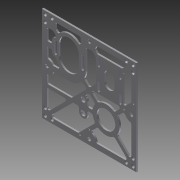
# Autodesk Inventor part: upper gearbox top plate
Saved by Autodesk Inventor 2012 (Build 160160000, 160)
## iProperties
Created: 2012-07-07
Part Number: upper gearbox top plate
Material: Default
Document SubType Name: Modeling
Designer: Bryce
Density: 1 g/cm^3
Author: Bryce
Autodesk Inventor part; units mm, degrees
ref_plane "YZ Plane" through (0, 0, 0) normal (1, 0, 0) x (0, 1, 0)
ref_plane "XZ Plane" through (0, 0, 0) normal (0, 1, 0) x (-1, 0, 0)
ref_plane "XY Plane" through (0, 0, 0) normal (0, 0, 1) x (1, 0, 0)
sketch "Sketch1" plane through (0, 0, 0) normal (0, 0, 1) x (1, 0, 0)
  line L0 (-114.3, 114.3) -> (63.5, 114.3)
  line L1 (63.5, 114.3) -> (63.5, -28.575)
  line L2 (63.5, -63.5) -> (28.575, -63.5)
  line L3 (-114.3, -63.5) -> (-114.3, 114.3)
  circle A0 centre (6.35, -6.35) radius 17.4625
  circle A1 centre (44.45, 107.95) radius 1.5875
  circle A2 centre (-95.25, -57.15) radius 1.5875
  circle A3 centre (-107.95, 95.25) radius 1.5875
  circle A4 centre (-107.95, 107.95) radius 1.5875
  circle A5 centre (-95.25, 107.95) radius 1.5875
  circle A6 centre (57.15, 95.25) radius 1.5875
  circle A7 centre (-107.95, -57.15) radius 1.5875
  circle A8 centre (-107.95, -44.45) radius 1.5875
  circle A9 centre (57.15, 107.95) radius 1.5875
  circle A10 centre (-63.5, 73.025) radius 19.05
  circle A11 centre (-63.5, 53.975) radius 19.05
  line L4 (-82.55, 73.025) -> (-44.45, 73.025)
  line L5 (-44.45, 73.025) -> (-44.45, 53.975)
  line L6 (-44.45, 53.975) -> (-82.55, 53.975)
  line L7 (-82.55, 53.975) -> (-82.55, 73.025)
  arc A12 (-13.7147, 9.2246) -> (-18.8508, -3.175) centre (6.35, -6.35) ccw
  arc A13 (26.4147, -21.9246) -> (26.4147, 9.2246) centre (6.35, -6.35) ccw
  arc A14 (-9.2246, -26.4147) -> (21.9246, -26.4147) centre (6.35, -6.35) ccw
  arc A15 (21.9246, 13.7147) -> (-9.2246, 13.7147) centre (6.35, -6.35) ccw
  arc A16 (-63.3483, 22.2254) -> (-38.6735, 34.1834) centre (-63.5, 53.975) ccw
  line L8 (53.975, 104.775) -> (53.975, 45.7651)
  line L9 (53.975, -53.975) -> (49.4849, -53.975) construction
  line L10 (-104.775, -53.975) -> (-104.775, -49.4849) construction
  line L11 (-63.3483, 22.2254) -> (-92.4782, 22.2254)
  line L12 (21.9246, -26.4147) -> (36.7849, -41.275)
  line L13 (26.4147, -21.9246) -> (41.275, -36.7849)
  line L14 (-13.7147, -21.9246) -> (-45.7651, -53.975)
  line L15 (-9.2246, -26.4147) -> (-24.1468, -41.337)
  line L16 (-13.7147, 9.2246) -> (-25.4, 20.9099)
  line L17 (-9.2246, 13.7147) -> (-20.9099, 25.4)
  line L18 (26.4147, 9.2246) -> (41.337, 24.1468)
  line L19 (21.9246, 13.7147) -> (36.7849, 28.575)
  arc A17 (-35.1635, 39.6536) -> (-31.75, 53.975) centre (-63.5, 53.975) ccw
  line L20 (53.975, -49.4849) -> (53.975, -53.975) construction
  line L21 (49.4849, -53.975) -> (36.7849, -53.975)
  line L22 (-45.7651, -53.975) -> (-100.2849, -53.975)
  line L23 (-104.775, -53.975) -> (-60.325, -9.525) construction
  line L24 (-104.775, -49.4849) -> (-64.8151, -9.525)
  line L25 (53.975, 104.775) -> (38.1, 88.9) construction
  line L26 (53.975, 100.2849) -> (38.1, 84.4099)
  line L27 (49.4849, 104.775) -> (36.7849, 92.075)
  line L28 (-58.4651, -3.175) -> (-29.8901, 25.4)
  line L29 (-29.8901, 25.4) -> (-38.6735, 34.1834)
  line L30 (-25.4, 29.8901) -> (-35.1635, 39.6536)
  line L31 (-18.8508, -3.175) -> (-28.751, -3.175)
  line L32 (-104.775, -9.525) -> (-64.8151, -9.525)
  line L33 (-58.4651, -3.175) -> (-104.775, -3.175)
  arc A18 (-18.8508, -9.525) -> (-13.7147, -21.9246) centre (6.35, -6.35) ccw
  line L34 (-55.8349, -9.525) -> (-100.2849, -53.975)
  line L35 (-49.4849, -3.175) -> (-34.0583, 12.2516) construction
  line L36 (36.7849, -53.975) -> (-12.7, -53.975)
  line L37 (53.975, -36.7849) -> (53.975, -49.4849)
  line L38 (41.275, -36.7849) -> (53.975, -49.4849)
  line L39 (36.7849, -41.275) -> (49.4849, -53.975)
  line L40 (28.575, -63.5) -> (-114.3, -63.5)
  line L41 (63.5, -28.575) -> (63.5, -63.5)
  line L42 (-25.4, -53.975) -> (-25.4, -63.5) construction
  circle A19 centre (44.45, -57.15) radius 1.5875
  circle A20 centre (57.15, -57.15) radius 1.5875
  circle A21 centre (57.15, -44.45) radius 1.5875
  line L43 (6.35, -6.35) -> (-25.0809, -37.7809) construction
  line L44 (-43.0414, -55.7414) -> (-50.8, -63.5) construction
  line L45 (-25.0809, -37.7809) -> (-43.0414, -55.7414) construction
  line L46 (6.35, -6.35) -> (40.026, 27.326) construction
  line L47 (40.026, 27.326) -> (57.9865, 45.2865) construction
  line L48 (57.9865, 45.2865) -> (63.5, 50.8) construction
  arc A22 (-12.7, -53.975) -> (-24.1468, -41.337) centre (-25.4, -53.975) ccw
  arc A23 (41.337, 24.1468) -> (53.975, 12.7) centre (53.975, 25.4) ccw
  line L49 (53.975, 12.7) -> (53.975, -36.7849)
  arc A24 (-31.75, 93.7765) -> (-19.808, 93.3724) centre (-25.4, 104.775) ccw
  line L50 (-31.75, 93.7765) -> (-31.75, 53.975)
  line L51 (-12.7, 104.775) -> (53.975, 104.775)
  arc A25 (-104.775, 12.7) -> (-92.4782, 22.2254) centre (-104.775, 25.4) ccw
  line L52 (-91.44, 53.975) -> (-86.36, 53.975)
  line L53 (-86.36, 53.975) -> (-86.36, 73.025)
  line L54 (-86.36, 73.025) -> (-91.44, 73.025)
  line L55 (-91.44, 73.025) -> (-91.44, 53.975)
  arc A26 (-86.36, 73.025) -> (-91.44, 73.025) centre (-88.9, 73.025) ccw
  arc A27 (-91.44, 53.975) -> (-86.36, 53.975) centre (-88.9, 53.975) ccw
  line L56 (-40.64, 53.975) -> (-35.56, 53.975)
  line L57 (-35.56, 53.975) -> (-35.56, 73.025)
  line L58 (-35.56, 73.025) -> (-40.64, 73.025)
  line L59 (-40.64, 73.025) -> (-40.64, 53.975)
  arc A28 (-35.56, 73.025) -> (-40.64, 73.025) centre (-38.1, 73.025) ccw
  arc A29 (-40.64, 53.975) -> (-35.56, 53.975) centre (-38.1, 53.975) ccw
  line L60 (-36.6885, -17.4625) -> (6.35, -6.35) construction
  line L61 (-36.6885, 4.7625) -> (6.35, -6.35) construction
  line L62 (6.35, -6.35) -> (-104.775, -6.35) construction
  arc A30 (-28.751, 4.7625) -> (-34.0583, 12.2516) centre (-36.6885, 4.7625) ccw
  line L63 (-28.751, 4.7625) -> (-28.751, -3.175)
  arc A31 (-44.626, -17.4625) -> (-28.751, -17.4625) centre (-36.6885, -17.4625) ccw
  line L64 (-44.626, -9.525) -> (-44.626, -17.4625)
  line L65 (-28.751, -17.4625) -> (-28.751, -9.525)
  line L66 (-55.8349, -9.525) -> (-44.626, -9.525)
  line L67 (-28.751, -9.525) -> (-18.8508, -9.525)
  line L68 (-28.751, -3.175) -> (-49.4849, -3.175) construction
  line L69 (-34.0583, 12.2516) -> (-25.4, 20.9099)
  arc A32 (-9.7028, 74.295) -> (-5.5372, 74.295) centre (-7.62, 74.295) ccw
  line L70 (-5.5372, 74.295) -> (-9.7028, 74.295)
  line L71 (-9.7028, 74.295) -> (-9.7028, 86.995)
  arc A33 (-5.5372, 86.995) -> (-9.7028, 86.995) centre (-7.62, 86.995) ccw
  circle A34 centre (12.7, 66.675) radius 9.525
  line L72 (3.175, 66.675) -> (22.225, 66.675)
  line L73 (22.225, 66.675) -> (22.225, 53.975)
  circle A35 centre (12.7, 53.975) radius 9.525
  line L74 (3.175, 53.975) -> (3.175, 66.675)
  line L75 (22.225, 53.975) -> (3.175, 53.975)
  line L76 (-9.7028, 86.995) -> (-5.5372, 86.995)
  line L77 (-5.5372, 86.995) -> (-5.5372, 74.295)
  line L78 (30.9372, 74.295) -> (30.9372, 86.995)
  arc A36 (35.1028, 86.995) -> (30.9372, 86.995) centre (33.02, 86.995) ccw
  line L79 (35.1028, 86.995) -> (35.1028, 74.295)
  line L80 (35.1028, 74.295) -> (30.9372, 74.295)
  arc A37 (30.9372, 74.295) -> (35.1028, 74.295) centre (33.02, 74.295) ccw
  line L81 (-9.7028, 33.655) -> (-9.7028, 46.355)
  arc A38 (-5.5372, 46.355) -> (-9.7028, 46.355) centre (-7.62, 46.355) ccw
  line L82 (-5.5372, 46.355) -> (-5.5372, 33.655)
  line L83 (-5.5372, 33.655) -> (-9.7028, 33.655)
  arc A39 (-9.7028, 33.655) -> (-5.5372, 33.655) centre (-7.62, 33.655) ccw
  line L84 (30.9372, 33.655) -> (30.9372, 46.355)
  arc A40 (35.1028, 46.355) -> (30.9372, 46.355) centre (33.02, 46.355) ccw
  line L85 (35.1028, 46.355) -> (35.1028, 33.655)
  line L86 (35.1028, 33.655) -> (30.9372, 33.655)
  arc A41 (30.9372, 33.655) -> (35.1028, 33.655) centre (33.02, 33.655) ccw
  line L87 (-12.7, 92.075) -> (-10.3326, 92.075) construction
  line L88 (38.1, 92.075) -> (38.1, 84.4099) construction
  line L89 (36.7849, 28.575) -> (-17.7349, 28.575)
  line L90 (-12.7, 92.075) -> (-12.7, 85.0797) construction
  line L91 (-25.4, 104.775) -> (12.7, 60.325) construction
  line L92 (38.1, 84.4099) -> (38.1, 29.8901)
  line L93 (36.7849, 92.075) -> (38.1, 92.075) construction
  line L94 (-19.808, 93.3724) -> (-12.7, 85.0797)
  line L95 (-14.9868, 97.5049) -> (-10.3326, 92.075)
  line L96 (-10.3326, 92.075) -> (36.7849, 92.075)
  line L97 (-12.7, 85.0797) -> (-12.7, 42.5901)
  arc A42 (-19.808, 93.3724) -> (-14.9868, 97.5049) centre (-25.4, 104.775) ccw construction
  arc A43 (-14.9868, 97.5049) -> (-12.7, 104.775) centre (-25.4, 104.775) ccw
  line L98 (-25.4, 29.8901) -> (-12.7, 42.5901)
  line L99 (-20.9099, 25.4) -> (-17.7349, 28.575)
  line L100 (36.7849, 28.575) -> (38.1, 29.8901) construction
  line L101 (38.1, 29.8901) -> (53.975, 45.7651)
  arc A44 (-88.1063, 47.6748) -> (-75.7974, 31.7504) centre (-63.5, 53.975) ccw
  line L102 (-75.7974, 31.7504) -> (-93.7767, 31.7504)
  arc A45 (-93.7767, 31.7504) -> (-104.775, 38.1) centre (-104.775, 25.4) ccw
  line L103 (-104.775, 38.1) -> (-104.775, 57.15)
  line L104 (-104.775, 57.15) -> (-95.25, 57.15)
  line L105 (-95.25, 57.15) -> (-95.25, 53.975)
  arc A46 (-95.25, 53.975) -> (-88.1063, 47.6748) centre (-88.9, 53.975) ccw
  line L106 (-104.775, 88.9) -> (-93.3901, 88.9)
  line L107 (-104.775, 88.9) -> (-104.775, 66.675)
  line L108 (-104.775, 66.675) -> (-95.25, 66.675)
  line L109 (-95.25, 66.675) -> (-95.25, 73.025)
  line L110 (-114.3, 114.3) -> (63.5, -63.5) construction
  arc A47 (-87.0446, 82.5545) -> (-88.1063, 79.3252) centre (-63.5, 73.025) ccw
  arc A48 (-88.1063, 79.3252) -> (-95.25, 73.025) centre (-88.9, 73.025) ccw
  line L111 (-93.3901, 88.9) -> (-87.0446, 82.5545)
  line L112 (-88.9, 104.775) -> (-88.9, 93.3901)
  line L113 (-88.9, 93.3901) -> (-83.8006, 88.2908)
  arc A49 (-41.275, 85.3217) -> (-83.8006, 88.2908) centre (-63.5, 73.025) ccw
  line L114 (-41.275, 85.3217) -> (-41.275, 104.775)
  line L115 (-88.9, 104.775) -> (-41.275, 104.775)
  line L116 (-104.775, -49.4849) -> (-104.775, 12.7)
  line L117 (-100.2849, -53.975) -> (-104.775, -53.975) construction
  point P0 (0, 0)
  point P1 (-88.9, 63.5)
  point P2 (-38.1, 63.5)
  point P3 (3.175, 60.325)
  point P4 (12.7, 66.675)
  dimension "d87" = 38.1
  dimension "d89" = 38.1
  dimension "d309" = 19.05
  dimension "d310" = 19.05
  dimension "d0" = 114.3
  dimension "d1" = 177.8
  dimension "d2" = 177.8
  dimension "d3" = 114.3
  dimension "d4" = 34.925
  dimension "d5" = 57.15
  dimension "d6" = 57.15
  dimension "d10" = 3.175
  dimension "d12" = 3.175
  dimension "d15" = 6.35
  dimension "d16" = 19.05
  dimension "d19" = 6.35
  dimension "d20" = 19.05
  dimension "d23" = 3.175
  dimension "d24" = 6.35
  dimension "d25" = 19.05
  dimension "d26" = 3.175
  dimension "d27" = 6.35
  dimension "d28" = 6.35
  dimension "d29" = 6.35
  dimension "d30" = 19.05
  dimension "d34" = 3.175
  dimension "d35" = 6.35
  dimension "d36" = 6.35
  dimension "d37" = 6.35
  dimension "d38" = 19.05
  dimension "d39" = 3.175
  dimension "d40" = 3.175
  dimension "d47" = 3.175
  dimension "d48" = 6.35
  dimension "d49" = 6.35
  dimension "d50" = 3.175
  dimension "d51" = 19.05
  dimension "d52" = 6.35
  dimension "d88" = 41.275
  dimension "d91" = 50.8
  dimension "d95" = 19.05
  dimension "d98" = 25.4
  dimension "d99" = 25.4
  dimension "d140" = 25.4
  dimension "d141" = 25.4
  dimension "d142" = 25.4
  dimension "d143" = 25.4
  dimension "d167" = 9.525
  dimension "d168" = 9.525
  dimension "d169" = 31.75
  dimension "d171" = 158.75
  dimension "d172" = 158.75
  dimension "d173" = 9.525
  dimension "d174" = 9.525
  dimension "d177" = 92.0746
  dimension "d180" = 45
  dimension "d182" = 6.35
  dimension "d183" = 6.35
  dimension "d186" = 6.35
  dimension "d188" = 6.35
  dimension "d190" = 3.175
  dimension "d195" = 3.175
  dimension "d197" = 3.175
  dimension "d198" = 6.35
  dimension "d204" = 3.175
  dimension "d205" = 3.175
  dimension "d206" = 6.35
  dimension "d207" = 3.175
  constraints: 238 end point, 71 point on circle, 70 parallel, 46 centre point, 42 perpendicular, 25 point on line, 21 coincident, 15 collinear, 13 tangent, 10 horizontal, 6 horizontal alignment, 4 midpoint, 4 vertical alignment, 3 symmetric about line, 3 vertical, 56 other
  measures "d0" distance from line of L0 point (0, 0)
  measures "d1" distance of L0.end L2.start
  measures "d2" distance of L0.start L0.end
  measures "d3" distance from line of L3 point (0, 0)
  measures "d4" diameter of A0
  measures "d5" distance from line of L1 A0.centre
  measures "d6" distance from line of L2 A0.centre
  measures "d10" diameter of A1
  measures "d12" diameter of A2
  measures "d15" distance from line of L0 A1.centre
  measures "d16" distance from line of L1 A1.centre
  measures "d19" distance from line of L2 A2.centre
  measures "d20" distance from line of L3 A2.centre
  measures "d23" diameter of A3
  measures "d24" distance from line of L3 A3.centre
  measures "d25" distance from line of L0 A3.centre
  measures "d26" diameter of A4
  measures "d27" distance from line of L0 A4.centre
  measures "d28" distance from line of L3 A4.centre
  measures "d29" distance from line of L0 A5.centre
  measures "d30" distance from line of L3 A5.centre
  measures "d34" diameter of A9
  measures "d35" distance from line of L0 A9.centre
  measures "d36" distance from line of L1 A9.centre
  measures "d37" distance from line of L1 A6.centre
  measures "d38" distance from line of L0 A6.centre
  measures "d39" diameter of A6
  measures "d40" diameter of A5
  measures "d47" diameter of A7
  measures "d48" distance from line of L2 A7.centre
  measures "d49" distance from line of L3 A7.centre
  measures "d50" diameter of A8
  measures "d51" distance from line of L2 A8.centre
  measures "d52" distance from line of L3 A8.centre
  measures "d88" distance from line of L0 point (-63.5, 73.025)
  measures "d91" distance from line of point (-63.5, 53.975) L3
  measures "d95" distance of L6.end L4.start
  measures "d98" horizontal distance of point (-63.5, 53.975) point (-88.9, 63.5)
  measures "d99" horizontal distance of point (-38.1, 63.5) point (-63.5, 73.025)
  measures "d140" radius of A13
  measures "d141" radius of A14
  measures "d142" radius of A12
  measures "d143" radius of A15
  measures "d167" distance from line of L4 point (-88.9, 63.5)
  measures "d168" distance from line of L4 point (-38.1, 63.5)
  measures "d169" radius of A16
  measures "d171" distance of L9.start L23.start
  measures "d172" distance of L8.start L9.start
  measures "d173" distance between parallel lines of L2 L9
  measures "d174" distance between parallel lines of L1 L8
  measures "d177" distance between parallel lines of L0 L11
  measures "d180" angle of L9 L12
  measures "d182" distance between parallel lines of L13 L12
  measures "d183" distance between parallel lines of L14 L15
  measures "d186" distance between parallel lines of L17 L16
  measures "d188" distance between parallel lines of L19 L18
  measures "d190" distance from line of L14 A0.centre
  measures "d195" distance between parallel lines of L24 L23
  measures "d197" distance between parallel lines of L27 L25
  measures "d198" distance between parallel lines of L26 L27
  measures "d204" distance from line of A0.centre L31
  measures "d205" distance from line of A0.centre L32
  measures "d206" distance between parallel lines of L32 L33
  measures "d207" distance between parallel lines of L34 L23
extrude "Extrusion8" add sketch "Sketch1" along normal blind 3.175 contours L0 L1 L41 L2 L40 L3 | L55 L54 L53 L52 | L52 A27 | A26 L54 | L59 L58 L57 L56 | L56 A29 | A28 L58 | L70 A32 | L71 L76 L77 L70 | A33 L76 | L72 A34 | L73 A35 A34 | A34 A35 L72 | A34 A35 L74 | A35 L75 A34 | A34 A35 | A35 L75 | L78 A36 L79 L80 | L80 A37 | L81 A38 L82 L83 | L83 A39 | L84 A40 L85 L86 | L86 A41 | A44 L102 A45 L103 L104 L105 A46 | L106 L111 A47 A48 L109 L108 L107 | L115 L114 A49 L113 L112
fillet "Fillet3" radius 3.175 31 edges at (21.9246, -26.4147, 1.5875) (49.4849, -53.975, 1.5875) (53.975, -49.4849, 1.5875) (-9.2246, -26.4147, 1.5875) (26.4147, 9.2246, 1.5875) (26.4147, -21.9246, 1.5875) (-18.8508, -9.525, 1.5875) (-9.2246, 13.7147, 1.5875) (21.9246, 13.7147, 1.5875) (-13.7147, -21.9246, 1.5875) (-45.7651, -53.975, 1.5875) (53.975, 45.7651, 1.5875) (-55.8349, -9.525, 1.5875) (-100.2849, -53.975, 1.5875) (53.975, 100.2849, 1.5875) (38.1, 84.4099, 1.5875) (-18.8508, -3.175, 1.5875) (-20.9099, 25.4, 1.5875) (-25.4, 20.9099, 1.5875) (-13.7147, 9.2246, 1.5875) (-104.775, -9.525, 1.5875) (-104.775, -49.4849, 1.5875) (-64.8151, -9.525, 1.5875) (36.7849, 92.075, 1.5875) (49.4849, 104.775, 1.5875) (-104.775, -3.175, 1.5875) (-58.4651, -3.175, 1.5875) (-29.8901, 25.4, 1.5875) (-38.6735, 34.1834, 1.5875) (-25.4, 29.8901, 1.5875) (-35.1635, 39.6536, 1.5875)
hole "Hole5" at (-88.9, 63.5, 0) at (-38.1, 63.5, 0) direction (0, 0, 1) diameter 5.08 end through all
hole "Hole6" at (-43.0414, -55.7414, 0) at (-25.0809, -37.7809, 0) direction (0, 0, 1) diameter 3.175 end through all
hole "Hole7" at (40.026, 27.326, 0) at (57.9865, 45.2865, 0) direction (0, 0, 1) diameter 3.175 end through all
chamfer "Chamfer1" distance 1.5875 angle 45 12 edges at (-109.5375, -57.15, 3.175) (-109.5375, -44.45, 3.175) (-96.8375, -57.15, 3.175) (42.8625, -57.15, 3.175) (55.5625, -57.15, 3.175) (55.5625, -44.45, 3.175) (55.5625, 95.25, 3.175) (55.5625, 107.95, 3.175) (42.8625, 107.95, 3.175) (-96.8375, 107.95, 3.175) (-109.5375, 107.95, 3.175) (-109.5375, 95.25, 3.175)
hole "Hole8" at (-25.4, -53.975, 0) at (53.975, 25.4, 0) at (-25.4, 104.775, 0) at (-104.775, 25.4, 0) direction (0, 0, 1) diameter 6.35 end through all
fillet "Fillet4" radius 3.175 8 edges at (-92.4782, 22.2254, 1.5875) (-104.775, 12.7, 1.5875) (-24.1468, -41.337, 1.5875) (-12.7, -53.975, 1.5875) (53.975, 12.7, 1.5875) (41.337, 24.1468, 1.5875) (-12.7, 104.775, 1.5875) (-31.75, 93.7765, 1.5875)
fillet "Fillet5" [suppressed]
extrude "Extrusion9" cut sketch "Sketch1" along normal blind 25.4 contours L55 L54 L53 L52 | L52 A27 | A26 L54 | L59 L58 L57 L56 | L56 A29 | A28 L58
fillet "Fillet6" radius 3.175 4 edges at (-34.0583, 12.2516, 1.5875) (-44.626, -9.525, 1.5875) (-28.751, -9.525, 1.5875) (-28.751, -3.175, 1.5875)
hole "Hole9" at (-36.6885, 4.7625, 0) at (-36.6885, -17.4625, 0) direction (0, 0, 1) diameter 9.2964 end through all
fillet "Fillet7" radius 3.175 8 edges at (36.7849, 28.575, 1.5875) (38.1, 29.8901, 1.5875) (-12.7, 85.0797, 1.5875) (-19.808, 93.3724, 1.5875) (-14.9868, 97.5049, 1.5875) (-10.3326, 92.075, 1.5875) (-12.7, 42.5901, 1.5875) (-17.7349, 28.575, 1.5875)
extrude "Extrusion10" cut sketch "Sketch1" along normal blind 25.4 contours L70 A32 | L71 L76 L77 L70 | A33 L76 | L72 A34 | L73 A35 A34 | A34 A35 L72 | A34 A35 L74 | A35 L75 A34 | A34 A35 | A35 L75 | L78 A36 L79 L80 | L80 A37 | L81 A38 L82 L83 | L83 A39 | L84 A40 L85 L86 | L86 A41
extrude "Extrusion11" cut sketch "Sketch1" along normal blind 25.4 contours A44 L102 A45 L103 L104 L105 A46 | L106 L111 A47 A48 L109 L108 L107 | L115 L114 A49 L113 L112
fillet "Fillet8" radius 3.175 17 edges at (-75.7974, 31.7504, 1.5875) (-93.7767, 31.7504, 1.5875) (-104.775, 38.1, 1.5875) (-104.775, 57.15, 1.5875) (-95.25, 57.15, 1.5875) (-88.1063, 47.6748, 1.5875) (-95.25, 66.675, 1.5875) (-104.775, 66.675, 1.5875) (-104.775, 88.9, 1.5875) (-93.3901, 88.9, 1.5875) (-88.9, 104.775, 1.5875) (-88.9, 93.3901, 1.5875) (-41.275, 104.775, 1.5875) (-41.275, 85.3217, 1.5875) (-87.0446, 82.5545, 1.5875) (-83.8006, 88.2908, 1.5875) (-88.1063, 79.3252, 1.5875)
equation "\"d89\" = d87"
body "Solid5"
